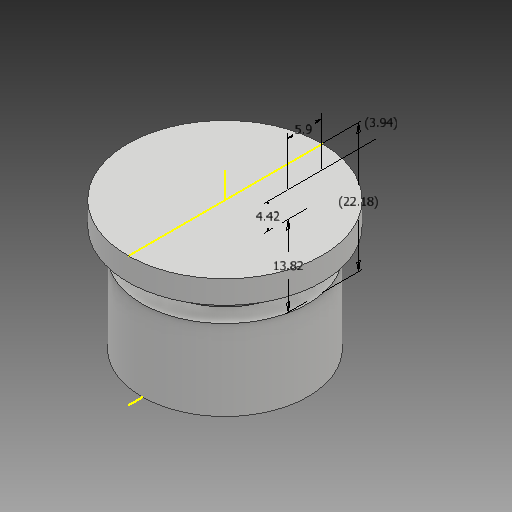
# Autodesk Inventor part: Pinion12T
Saved by Autodesk Inventor 2019.2 (Build 232265000, 265)
## iProperties
Created: 2017-11-17
Part Number: Pinion12T
Material: Generic
Document SubType Name: Modeling
Designer: eroldan
Density: 1 g/cm^3
Appearance: Default
Author: eroldan
Autodesk Inventor part; units mm, degrees
ref_plane "YZ Plane" through (0, 0, 0) normal (1, 0, 0) x (0, 1, 0)
ref_plane "XZ Plane" through (0, 0, 0) normal (0, 1, 0) x (-1, 0, 0)
ref_plane "XY Plane" through (0, 0, 0) normal (0, 0, 1) x (1, 0, 0)
sketch "Sketch1" plane through (0, 0, 0) normal (0, 0, 1) x (1, 0, 0)
  circle A0 centre (0, 0) radius 16.65
  dimension "d0" = 33.3
  constraints: 1 centre point, 1 coincident
  measures "d0" diameter of A0
extrude "Extrusion1" add sketch "Sketch1" along normal blind 22.18
sketch "Sketch2" plane through (0, 0, 0) normal (1, 0, 0) x (0, 1, 0)
  line L0 (14.2427, 0) -> (14.2427, 13.82)
  line L1 (14.2427, 13.82) -> (10.75, 13.82)
  line L2 (10.75, 13.82) -> (10.75, 18.24)
  line L3 (10.75, 18.24) -> (16.65, 18.24)
  line L4 (16.65, 0) -> (16.65, 22.18) projected
  line L5 (-16.65, 0) -> (16.65, 0) projected
  line L6 (14.2427, 0) -> (16.65, 0)
  line L7 (16.65, 0) -> (16.65, 18.24)
  line L8 (0, -4.436) -> (0, 26.616) projected
  line L9 (16.65, 22.18) -> (-16.65, 22.18) projected
  point P0 (0, 0)
  dimension "d3" = 13.82
  dimension "d4" = 4.42
  dimension "d5" = 5.9
  dimension "d7" = 22.18
  dimension "d8" = 3.94
  constraints: 12 end point, 3 perpendicular, 1 collinear, 1 horizontal, 1 point on line, 1 vertical
  measures "d3" distance of L0.start L0.end
  measures "d4" distance of L1.end L2.end
  measures "d5" distance of L2.end L3.end
  measures "d7" distance between parallel lines of L5 L9
  measures "d8" distance from line of L2.end L9
revolve "Revolution1" cut sketch "Sketch2" angle 360 about axis through (0, 0, -10) along (0, 0, 1) contours L0 L1 L2 L3 L4 L5
body "Solid1"
